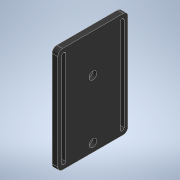
# Autodesk Inventor part: 24_Laserholder
Saved by Autodesk Inventor 2022.2 (Build 262287010, 287A)
## iProperties
Created: 2022-05-02
Part Number: 24_Laserholder
Material: PET-Kunststoff
Document SubType Name: Modeling
Designer: MXBD
Density: 1.541 g/cm^3
Appearance: Gummi - Schwarz
Author: MXBD
Autodesk Inventor part; units mm, degrees
ref_plane "YZ Plane" through (0, 0, 0) normal (1, 0, 0) x (0, 1, 0)
ref_plane "XZ Plane" through (0, 0, 0) normal (0, 1, 0) x (-1, 0, 0)
ref_plane "XY Plane" through (0, 0, 0) normal (0, 0, 1) x (1, 0, 0)
sketch "Skizze1" plane through (0, 0, 0) normal (1, 0, 0) x (0, 1, 0)
  line L0 (-63, 0) -> (63, 0) projected
  line L1 (0, 42) -> (0, -42) projected
  line L2 (-45, 30) -> (45, 30)
  line L3 (45, 30) -> (45, -30)
  line L4 (45, -30) -> (-45, -30)
  line L5 (-45, -30) -> (-45, 30)
  line L6 (-45, 30) -> (45, -30) construction
  line L7 (45, 30) -> (-45, -30) construction
  point P0 (0, 0)
  dimension "d21" = 90
  dimension "d22" = 60
  constraints: 12 end point, 4 midpoint, 2 parallel, 1 horizontal, 1 perpendicular
  measures "d21" distance of L3.end L4.end
  measures "d22" distance of L2.end L3.end
extrude "Extrusion1" add sketch "Skizze1" along normal mid plane 5
sketch "Skizze2" plane through (2.5, 0, 0) normal (1, 0, 0) x (0, 0, -1)
  line L0 (-42, 0) -> (42, 0) projected
  line L1 (0, -63) -> (0, 63) projected
  line L2 (-30, -45) -> (30, -45) projected
  point P0 (0, 0)
  point P1 (0, 12)
  point P2 (0, -38)
  dimension "d23" = 50
  dimension "d24" = 7
  constraints: 2 point on line
  measures "d23" distance of point (0, -38) point (0, 12)
  measures "d24" distance from line of L2 point (0, -38)
hole "Bohrung1" at (2.5, -38, 0) at (2.5, 12, 0) direction (-1, 0, 0) diameter 3.4 end through all counterbore diameter 6.5 counterbore depth 3.4 clearance for "Inbusschraube ISO 4762" size "M3" standard "ISO"
sketch "Skizze3" plane through (2.5, 0, 0) normal (1, 0, 0) x (0, 0, -1)
  line L0 (0, -63) -> (0, 63) projected
  line L1 (-42, 0) -> (42, 0) projected
  line L2 (-25, -40) -> (-25, 40) construction
  line L3 (-23.35, -40) -> (-23.35, 40)
  line L4 (-26.65, 40) -> (-26.65, -40)
  arc A0 (-26.65, -40) -> (-23.35, -40) centre (-25, -40) ccw
  arc A1 (-23.35, 40) -> (-26.65, 40) centre (-25, 40) ccw
  point P0 (0, 0)
  point P1 (-25, 0)
  point P2 (-26.65, 0)
  point P3 (-23.35, 0)
  dimension "d14" = 3.3
  dimension "d15" = 80
  dimension "d16" = 25
  constraints: 8 end point, 4 point on circle, 4 tangent, 2 centre point, 1 midpoint, 1 parallel, 1 perpendicular, 1 point on line
  measures "d14" diameter of A1
  measures "d15" distance of L2.start L2.end
  measures "d16" distance from line of L0 point (-25, 0)
extrude "Extrusion2" cut sketch "Skizze3" against normal through all
mirror "Spiegeln1" about plane through (0, 0, 0) normal (0, 0, 1) of "Extrusion2"
fillet "Rundung1" radius 4 4 edges at (0, 45, 30) (0, 45, -30) (0, -45, 30) (0, -45, -30)
